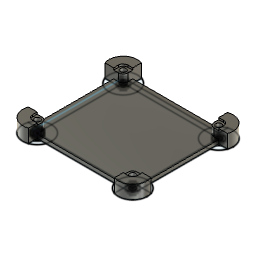
orangeBox (Autodesk Fusion 360 design; units mm, degrees)
Autodesk Fusion 360 part; units mm, degrees
note: some values were not read from the file. Set by a fixed rule: which sketch regions a step uses.
sketch "Sketch1" plane through (0, 0, 0) normal (0, 0, 1) x (1, 0, 0)
  line L0 (0, 0) -> (60, 0)
  line L1 (60, 0) -> (60, 60)
  line L2 (60, 60) -> (0, 60)
  line L3 (0, 60) -> (0, 0)
  line L4 (2, 2) -> (58, 2)
  line L5 (58, 2) -> (58, 58)
  line L6 (58, 58) -> (2, 58)
  line L7 (2, 58) -> (2, 2)
  dimension "d1" = 60
  dimension "d2" = 60
  dimension "d3" = 56
  dimension "d4" = 56
  constraint horizontal L0
  constraint vertical L1
  constraint horizontal L2
  constraint vertical L3
  constraint coincident L0.start L3.end
  constraint horizontal L4
  constraint vertical L5
  constraint horizontal L6
  constraint vertical L7
  measures "d1" distance of L0.start L0.end
  measures "d2" distance of L0.start L2.end
  measures "d3" distance of L4.start L4.end
  measures "d4" distance of L4.start L6.end
sketch "Sketch2" plane through (0, 0, 2) normal (0, 0, 1) x (-1, 0, 0)
  line L0 (-2, -2) -> (-4.5, -2)
  line L1 (-4.5, -2) -> (-4.5, -5)
  line L2 (-4.5, -5) -> (-2, -5)
  line L3 (-2, -5) -> (-2, -2)
  line L4 (-2, -58) -> (-4.5, -58)
  line L5 (-4.5, -58) -> (-4.5, -55)
  line L6 (-4.5, -55) -> (-2, -55)
  line L7 (-2, -55) -> (-2, -58)
  line L8 (-58, -58) -> (-49.5, -58)
  line L9 (-49.5, -58) -> (-49.5, -55)
  line L10 (-49.5, -55) -> (-58, -55)
  line L11 (-58, -55) -> (-58, -58)
  line L12 (-58, -2) -> (-49.5, -2)
  line L13 (-49.5, -2) -> (-49.5, -5)
  line L14 (-49.5, -5) -> (-58, -5)
  line L15 (-58, -5) -> (-58, -2)
  circle A0 centre (-4.5, -55) radius 1
  circle A1 centre (-49.5, -55) radius 1
  circle A2 centre (-4.5, -5) radius 1
  circle A3 centre (-49.5, -5) radius 1
  line L16 (-2, -58) -> (-2, -2)
  line L17 (-2, -2) -> (-58, -2)
  line L18 (-58, -2) -> (-58, -58)
  line L19 (-58, -58) -> (-2, -58)
  dimension "d9" = 2.5
  dimension "d10" = 3
  dimension "d11" = 2.5
  dimension "d12" = 3
  dimension "d13" = 8.5
  dimension "d14" = 3
  dimension "d15" = 8.5
  dimension "d16" = 3
  dimension "d17" = 2
  dimension "d18" = 2
  dimension "d19" = 2
  dimension "d20" = 2
  constraint horizontal L0
  constraint vertical L1
  constraint horizontal L2
  constraint vertical L3
  constraint horizontal L4
  constraint vertical L5
  constraint horizontal L6
  constraint vertical L7
  constraint horizontal L8
  constraint vertical L9
  constraint horizontal L10
  constraint vertical L11
  constraint horizontal L12
  constraint vertical L13
  constraint horizontal L14
  constraint vertical L15
  constraint coincident L5.end L6.start
  constraint coincident L9.end L10.start
  constraint coincident L1.end L2.start
  constraint coincident L13.end L14.start
  measures "d9" distance of L0.start L0.end
  measures "d10" distance of L0.start L2.end
  measures "d11" distance of L4.start L4.end
  measures "d12" distance of L4.start L6.end
  measures "d13" distance of L8.start L8.end
  measures "d14" distance of L8.start L10.end
  measures "d15" distance of L12.start L12.end
  measures "d16" distance of L12.start L14.end
  measures "d17" diameter of A0
  measures "d18" diameter of A1
  measures "d19" diameter of A2
  measures "d20" diameter of A3
sketch "Sketch3" plane through (0, 0, 0) normal (0, 0, 1) x (1, 0, 0)
  circle A0 centre (0, 45) radius 1.5
  circle A1 centre (50, 45) radius 1.5
  circle A2 centre (50, 0) radius 1.5
  circle A3 centre (0, 0) radius 1.5
  line L0 (0, -2.5) -> (50, -2.5)
  line L1 (52.5, 0) -> (52.5, 45)
  line L2 (-2.5, 0.0027) -> (-2.5, 45)
  line L3 (0.0001, 47.5) -> (50, 47.5)
  circle A4 centre (0, 45) radius 7.5
  circle A5 centre (0, 0) radius 7.5
  circle A6 centre (50, 45) radius 7.5
  circle A7 centre (50, 0) radius 7.5
  line L4 (0, 42.5) -> (-7.0711, 42.5)
  line L5 (2.5, 45) -> (2.5, 52.0711)
  line L6 (47.5, 45) -> (47.5, 52.0711)
  line L7 (50, 42.5) -> (57.0711, 42.5)
  line L8 (50, 2.5) -> (57.0711, 2.5)
  line L9 (47.5, 0) -> (47.5, -7.0711)
  line L10 (0, 2.5) -> (-7.0711, 2.5)
  line L11 (2.5, 0) -> (2.5, -7.0711)
  arc A8 (0, 42.5) -> (2.5, 45) centre (0, 45) ccw
  arc A9 (0.0001, 47.5) -> (-2.5, 45) centre (0, 45) ccw
  line L12 (0, 45) -> (0, 43.5)
  line L13 (1.5, 45) -> (0, 45)
  arc A10 (47.5, 45) -> (50, 42.5) centre (50, 45) ccw
  arc A11 (52.5, 45) -> (50, 47.5) centre (50, 45) ccw
  line L14 (50, 43.5) -> (50, 45)
  line L15 (50, 45) -> (48.5, 45)
  line L16 (47.5, 45) -> (2.5, 45)
  arc A12 (50, 2.5) -> (47.5, 0) centre (50, 0) ccw
  arc A13 (50, -2.5) -> (52.5, 0) centre (50, 0) ccw
  line L17 (48.5, 0) -> (50, 0)
  line L18 (50, 0) -> (50, 1.5)
  line L19 (50, 2.5) -> (50, 42.5)
  arc A14 (-2.5, 0.0027) -> (0, -2.5) centre (0, 0) ccw
  arc A15 (2.5, 0) -> (0, 2.5) centre (0, 0) ccw
  line L20 (0, 0) -> (1.5, 0)
  line L21 (2.5, 0) -> (47.5, 0)
  line L22 (0, 42.5) -> (0, 2.5)
  line L23 (0, 1.5) -> (0, 0)
  dimension "d23" = 50
  dimension "d24" = 45
  dimension "d25" = 3
  dimension "d26" = 3
  dimension "d27" = 3
  dimension "d28" = 3
  dimension "d29" = 5
  dimension "d30" = 5
  dimension "d31" = 5
  dimension "d32" = 5
  dimension "d37" = 15
  dimension "d38" = 15
  dimension "d39" = 15
  dimension "d40" = 15
  constraint horizontal L20
  constraint vertical L18
  constraint horizontal L15
  constraint vertical L12
  constraint coincident A3.centre A5.centre
  constraint coincident A0.centre A4.centre
  constraint coincident A1.centre A6.centre
  constraint coincident A2.centre A7.centre
  constraint concentric A0 A8
  constraint concentric A1 A10
  constraint concentric A2 A12
  constraint coincident L0.end A12
  constraint tangent L0 A12
  constraint perpendicular L0 L12
  constraint coincident L1.end A10
  constraint tangent L1 A10
  constraint perpendicular L0 L1
  constraint tangent L2 A8
  constraint coincident L3.start A8
  constraint tangent L3 A10
  constraint concentric A0 A4
  constraint concentric A1 A6
  constraint concentric A7 A12
  constraint coincident L4.start L12
  constraint coincident A4 L4.end
  constraint tangent L4 A8
  constraint coincident A4 L5.end
  constraint tangent L5 A8
  constraint coincident L6.start L15
  constraint coincident A6 L6.end
  constraint tangent L6 A10
  constraint perpendicular L3 L6
  constraint coincident A6 L7.end
  constraint tangent L7 A10
  constraint coincident L8.start L18
  constraint coincident A7 L8.end
  constraint tangent L8 A12
  constraint coincident A7 L9.end
  constraint tangent L9 A12
  constraint coincident L10.start L12
  constraint coincident A5 L10.end
  constraint tangent L10 A14
  constraint coincident L11.start A14
  constraint coincident L11.start L20
  constraint coincident A5 L11.end
  constraint tangent L11 A14
  constraint concentric A8 A9
  constraint coincident A0 L12.end
  constraint collinear L12 L22
  constraint coincident A0 L13.start
  constraint collinear L13 L15
  constraint concentric A10 A11
  constraint coincident A1 L14.start
  constraint collinear L14 L18
  constraint coincident A1 L15.end
  constraint collinear L15 L16
  constraint concentric A12 A13
  constraint coincident A2 L17.start
  constraint collinear L17 L20
  constraint coincident A2 L18.end
  constraint collinear L18 L19
  constraint concentric A14 A15
  constraint coincident A3 L20.end
  constraint collinear L20 L21
  constraint coincident A3 L23.start
  constraint collinear L22 L23
  measures "d23" distance of A3.centre A2.centre
  measures "d24" distance of A3.centre A0.centre
  measures "d25" diameter of A0
  measures "d26" diameter of A1
  measures "d27" diameter of A2
  measures "d28" diameter of A3
  measures "d29" diameter of A14
  measures "d30" diameter of A8
  measures "d31" diameter of A10
  measures "d32" diameter of A12
  measures "d37" diameter of A4
  measures "d38" diameter of A5
  measures "d39" diameter of A6
  measures "d40" diameter of A7
extrude "Extrude6" add sketch "Sketch3" along normal blind 7 contours L0 L2 A5 L10 L11 A14 | L0 L1 A7 L8 L9 A13 | L2 L3 A4 L4 L5 A9 | L1 L3 A6 L6 L7 A11 makes body 1 at (48.1731, 52.2741, 2.3333) makes body 2 at (48.8622, -7.4132, 4.6667) makes body 3 at (-7.4132, 43.8622, 2.3333) makes body 4 at (2.1658, -7.1805, 4.6667)
extrude "Extrude7" add sketch "Sketch3" along normal blind 2 separate body contours L0 A5 L11 L21 | L0 A5 A7 L21 | A5 A15 L21 L22 | L2 A5 L10 L22 | L0 A7 L9 L21 | A4 A5 A6 A7 L16 L19 L21 L22 | L2 A4 A5 L22 | A7 A12 L19 L21 | L2 A4 L4 L22 | L1 A6 A7 L19 | L1 A7 L8 L19 | A4 A8 L16 L22 | L1 A6 L7 L19 | A6 A10 L16 L19 | L3 A4 L5 L16 | L3 A4 A6 L16 | L3 A6 L6 L16 makes body 5
extrude "Extrude8" add sketch "Sketch3" along normal blind 6 contours L0 L2 L10 L11 A14 A15 | L0 L1 L8 L9 A12 A13 | L2 L3 L4 L5 A8 A9 | L1 L3 L6 L7 A10 A11 bodies 1 2 3 4 5
